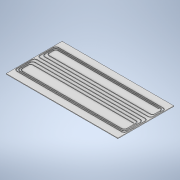
# Autodesk Inventor part: coil_layer
Saved by Autodesk Inventor 2021 (Build 250183000, 183)
## iProperties
Created: 2021-02-03
Part Number: coil_layer
Material: Generic
Document SubType Name: Modeling
Designer: User
Density: 1 g/cm^3
Appearance: Default
Author: User
Autodesk Inventor part; units mm, degrees
ref_plane "YZ Plane" through (0, 0, 0) normal (1, 0, 0) x (0, 1, 0)
ref_plane "XZ Plane" through (0, 0, 0) normal (0, 1, 0) x (-1, 0, 0)
ref_plane "XY Plane" through (0, 0, 0) normal (0, 0, 1) x (1, 0, 0)
sketch "Sketch1" plane through (0, 0, 0) normal (0, 1, 0) x (-1, 0, 0)
  line L0 (-17.9221, -19.934) -> (-497.9003, -19.934)
  line L1 (-517.9003, 3.6211) -> (-517.9003, 130.008)
  line L2 (-498.4559, 150) -> (251.5573, 150)
  line L3 (272.0997, 130.0022) -> (272.0997, 30.0874)
  line L4 (-18.4221, -15.434) -> (-497.9003, -15.434)
  line L5 (-513.4003, 3.3566) -> (-513.4003, 129.9936)
  line L6 (-498.4133, 145.5) -> (251.5937, 145.5)
  line L7 (267.5997, 130.0175) -> (267.5997, 30.093)
  line L8 (251.5818, 7.666) -> (-487.4606, 7.666)
  line L9 (-503.9003, 29.6772) -> (-503.9003, 120.4936)
  line L10 (251.5679, 3.166) -> (-477.2003, 3.166)
  line L11 (-508.4003, 30.3457) -> (-508.4003, 120.508)
  line L12 (-488.9133, 136) -> (242.0937, 136)
  line L13 (-488.9559, 140.5) -> (242.0573, 140.5)
  line L14 (258.0997, 120.5175) -> (258.0997, 56.5584)
  line L15 (242.2252, 30.766) -> (-474.4003, 30.766)
  line L16 (262.5997, 120.5022) -> (262.5997, 56.5974)
  line L17 (242.1573, 26.266) -> (-474.4003, 26.266)
  line L18 (-494.4003, 56.1758) -> (-494.4003, 110.9936)
  line L19 (-479.4133, 126.5) -> (232.5937, 126.5)
  line L20 (248.5997, 111.0175) -> (248.5997, 81.7203)
  line L21 (226.7413, 53.866) -> (-488.9221, 53.866)
  line L22 (-498.9003, 56.8436) -> (-498.9003, 111.008)
  line L23 (-479.4559, 131) -> (232.5573, 131)
  line L24 (253.0997, 111.0022) -> (253.0997, 83.0316)
  line L25 (226.7413, 49.366) -> (-488.9221, 49.366)
  line L26 (-122.9221, 150) -> (-122.9221, -150) construction
  line L27 (-18.9221, -15.434) -> (252.6121, -15.434)
  line L28 (271.0123, -33.8341) -> (271.0123, -129.4993)
  line L29 (251.5773, -149.4789) -> (-498.4319, -149.4789)
  line L30 (-518.377, -129.4966) -> (-518.377, -58.4688)
  line L31 (-18.9221, -19.934) -> (252.6121, -19.934)
  line L32 (266.5123, -33.8341) -> (266.5123, -129.4991)
  line L33 (251.5771, -144.9789) -> (-498.4273, -144.9789)
  line L34 (-498.449, -38.534) -> (242.0875, -38.534)
  line L35 (262.0712, -58.5177) -> (262.0712, -119.9846)
  line L36 (242.0769, -139.9789) -> (-488.9319, -139.9789)
  line L37 (-513.877, -129.4966) -> (-513.877, -58.4772)
  line L38 (-498.4397, -43.034) -> (242.0875, -43.034)
  line L39 (257.5712, -58.5177) -> (257.5712, -119.9846)
  line L40 (242.0769, -135.4789) -> (-488.9272, -135.4789)
  line L41 (-504.377, -119.9952) -> (-504.377, -84.5371)
  line L42 (-508.877, -119.9952) -> (-508.877, -84.9593)
  line L43 (-488.877, -61.634) -> (232.6078, -61.634)
  line L44 (252.6078, -84.9536) -> (252.6078, -110.5)
  line L45 (-488.877, -66.134) -> (232.6078, -66.134)
  line L46 (248.1078, -94.2732) -> (248.1078, -110.5)
  line L47 (232.5783, -125.9789) -> (-488.9221, -125.9789)
  line L48 (232.5775, -130.4789) -> (-488.9221, -130.4789)
  line L49 (-522.9003, 200.5211) -> (277.0997, 200.5211)
  arc A0 (251.5773, -149.4789) -> (271.0123, -129.4993) centre (251.2071, -129.6765) ccw
  arc A1 (251.5771, -144.9789) -> (266.5123, -129.4991) centre (251.2071, -129.6772) ccw
  arc A2 (242.0769, -135.4789) -> (257.5712, -119.9846) centre (242.0769, -119.9846) ccw
  arc A3 (242.0769, -139.9789) -> (262.0712, -119.9846) centre (242.0769, -119.9846) ccw
  arc A4 (232.5775, -130.4789) -> (252.6078, -110.5) centre (232.6051, -110.4763) ccw
  arc A5 (232.5783, -125.9789) -> (248.1078, -110.5) centre (232.6051, -110.4763) ccw
  line L50 (266.0656, -58.5177) -> (242.0875, -58.5177) construction
  line L51 (242.0875, -58.5177) -> (242.0875, -27) construction
  arc A6 (257.5712, -58.5177) -> (242.0875, -43.034) centre (242.0875, -58.5177) ccw
  arc A7 (262.0712, -58.5177) -> (242.0875, -38.534) centre (242.0875, -58.5177) ccw
  line L52 (252.6121, -3.7302) -> (252.6121, -33.8341) construction
  line L53 (252.6121, -33.8341) -> (272.6377, -33.8341) construction
  arc A8 (266.5123, -33.8341) -> (252.6121, -19.934) centre (252.6121, -33.8341) ccw
  arc A9 (271.0123, -33.8341) -> (252.6121, -15.434) centre (252.6121, -33.8341) ccw
  arc A10 (-518.377, -129.4966) -> (-498.4319, -149.4789) centre (-498.3932, -129.4952) ccw
  arc A11 (-513.877, -129.4966) -> (-498.4273, -144.9789) centre (-498.3932, -129.4952) ccw
  arc A12 (-508.877, -119.9952) -> (-488.9319, -139.9789) centre (-488.8932, -119.9952) ccw
  line L54 (-488.9221, -130.4789) -> (-488.9221, -125.9789)
  arc A13 (-504.377, -119.9952) -> (-488.9272, -135.4789) centre (-488.8932, -119.9952) ccw
  arc A14 (-498.4397, -43.034) -> (-513.877, -58.4772) centre (-498.3717, -58.5393) ccw
  arc A15 (-498.449, -38.534) -> (-518.377, -58.4688) centre (-498.3717, -58.5393) ccw
  line L55 (-488.9221, 49.366) -> (-488.9221, 53.866)
  arc A16 (-479.4133, 126.5) -> (-494.4003, 110.9936) centre (-479.0257, 111.1296) ccw
  arc A17 (-479.4559, 131) -> (-498.9003, 111.008) centre (-479.0257, 111.1296) ccw
  arc A18 (-488.9133, 136) -> (-503.9003, 120.4936) centre (-488.5257, 120.6296) ccw
  arc A19 (-488.9559, 140.5) -> (-508.4003, 120.508) centre (-488.5257, 120.6296) ccw
  arc A20 (-498.4133, 145.5) -> (-513.4003, 129.9936) centre (-498.0257, 130.1296) ccw
  arc A21 (-498.4559, 150) -> (-517.9003, 130.008) centre (-498.0257, 130.1296) ccw
  arc A22 (248.5997, 111.0175) -> (232.5937, 126.5) centre (232.9624, 110.8664) ccw
  arc A23 (253.0997, 111.0022) -> (232.5573, 131) centre (232.9624, 110.8664) ccw
  arc A24 (258.0997, 120.5175) -> (242.0937, 136) centre (242.4624, 120.3664) ccw
  arc A25 (262.5997, 120.5022) -> (242.0573, 140.5) centre (242.4624, 120.3664) ccw
  arc A26 (267.5997, 130.0175) -> (251.5937, 145.5) centre (251.9624, 129.8664) ccw
  arc A27 (272.0997, 130.0022) -> (251.5573, 150) centre (251.9624, 129.8664) ccw
  line L56 (-522.9003, -199.4789) -> (-522.9003, 200.5211)
  line L57 (267.5997, 30.093) -> (267.5997, 7.666) construction
  line L58 (267.5997, 7.666) -> (251.5818, 7.666) construction
  line L59 (242.1573, 26.266) -> (242.5997, 26.266) construction
  line L60 (262.5997, 26.266) -> (262.5997, 56.5974) construction
  line L61 (258.0997, 56.5584) -> (258.0997, 42.8204) construction
  line L62 (233.0997, 49.366) -> (253.0997, 49.366) construction
  line L63 (253.0997, 49.366) -> (253.0997, 83.0316) construction
  line L64 (248.5997, 81.7203) -> (248.5997, 53.866) construction
  line L65 (248.5997, 53.866) -> (232.2009, 53.866) construction
  line L66 (-494.4003, 56.1758) -> (-494.4003, 46.266) construction
  line L67 (-478.9003, 30.766) -> (-477.2003, 30.766) construction
  line L68 (-479.5767, 26.266) -> (-498.9003, 26.266) construction
  line L69 (-498.9003, 49.366) -> (-498.9003, 56.8436) construction
  line L70 (-487.4606, 7.666) -> (-503.9003, 7.666) construction
  line L71 (-503.9003, 29.6772) -> (-503.9003, 7.666) construction
  line L72 (-508.4003, 30.3457) -> (-508.4003, 23.166) construction
  line L73 (-508.4003, 3.166) -> (-489.0292, 3.166) construction
  line L74 (-498.4417, -15.434) -> (-513.4003, -15.434) construction
  line L75 (-517.9003, -19.934) -> (-498.4419, -19.934) construction
  line L76 (248.1078, -84.54) -> (248.1078, -66.134) construction
  line L77 (248.1078, -66.134) -> (232.6078, -66.134) construction
  line L78 (232.6078, -61.634) -> (252.6078, -61.634) construction
  line L79 (252.6078, -61.634) -> (252.6078, -84.9536) construction
  line L80 (-488.877, -61.634) -> (-508.877, -61.634) construction
  line L81 (-508.877, -61.634) -> (-508.877, -84.9593) construction
  line L82 (-488.877, -66.134) -> (-504.377, -66.134) construction
  line L83 (-504.377, -66.134) -> (-504.377, -84.5371) construction
  line L84 (-508.877, -61.634) -> (-508.877, -84.9593) construction
  line L85 (-498.9003, 26.266) -> (-488.9221, 26.266) construction
  line L86 (-478.9003, 26.266) -> (-478.9003, 46.266) construction
  line L87 (-478.9003, 46.266) -> (-498.9003, 46.266) construction
  line L88 (-494.4003, 50.766) -> (-494.4003, 46.266) construction
  line L89 (-474.4003, 30.766) -> (-474.4003, 26.266) construction
  arc A28 (-498.9003, 46.266) -> (-478.9003, 26.266) centre (-478.9003, 46.266) ccw
  arc A29 (-494.4003, 46.266) -> (-478.9003, 30.766) centre (-478.9003, 46.266) ccw
  line L90 (-498.9003, 56.8436) -> (-498.9003, 46.266)
  line L91 (-494.4003, 56.1758) -> (-494.4003, 46.266)
  line L92 (-478.9003, 30.766) -> (-474.4003, 30.766)
  line L93 (-478.9003, 26.266) -> (-474.4003, 26.266)
  line L94 (-488.4003, 3.166) -> (-488.4003, 23.166) construction
  line L95 (-488.4003, 23.166) -> (-508.4003, 23.166) construction
  arc A30 (-503.9003, 23.166) -> (-488.4003, 7.666) centre (-488.4003, 23.166) ccw
  line L96 (-488.4003, 7.666) -> (-487.4606, 7.666)
  line L97 (-477.2003, 9.3706) -> (-477.2003, 0.2696) construction
  arc A31 (-508.4003, 23.166) -> (-488.4003, 3.166) centre (-488.4003, 23.166) ccw
  line L98 (-508.4003, 30.3457) -> (-508.4003, 23.166)
  line L99 (-503.9003, 29.6772) -> (-503.9003, 23.166)
  line L100 (-488.4003, 3.166) -> (-477.2003, 3.166)
  line L101 (226.7413, 56.1758) -> (226.7413, 43.6622) construction
  arc A32 (233.0997, 53.866) -> (248.5997, 69.366) centre (233.0997, 69.366) ccw
  arc A33 (233.0997, 49.366) -> (253.0997, 69.366) centre (233.0997, 69.366) ccw
  line L102 (233.0997, 53.866) -> (226.7413, 53.866)
  line L103 (233.0997, 49.366) -> (226.7413, 49.366) construction
  line L104 (233.0997, 49.366) -> (226.7413, 49.366)
  line L105 (248.5997, 69.366) -> (248.5997, 81.7203)
  line L106 (253.0997, 83.0316) -> (253.0997, 69.366)
  line L107 (242.5997, 29.7117) -> (242.5997, 46.266) construction
  line L108 (242.5997, 46.266) -> (262.5997, 46.266) construction
  line L109 (242.1573, 26.266) -> (242.5997, 26.266) construction
  line L110 (242.1573, 26.266) -> (242.5997, 26.266)
  arc A34 (242.5997, 30.766) -> (258.0997, 46.266) centre (242.5997, 46.266) ccw
  arc A35 (242.5997, 26.266) -> (262.5997, 46.266) centre (242.5997, 46.266) ccw
  line L111 (258.0997, 46.266) -> (258.0997, 56.5584)
  line L112 (262.5997, 56.5974) -> (262.5997, 46.266)
  line L113 (242.2252, 30.766) -> (242.5997, 30.766)
  arc A36 (252.0997, 7.666) -> (267.5997, 23.166) centre (252.0997, 23.166) ccw
  line L114 (252.0997, 7.666) -> (251.5818, 7.666)
  line L115 (267.5997, 23.166) -> (267.5997, 30.093)
  arc A37 (252.0997, 3.166) -> (272.0997, 23.166) centre (252.0997, 23.166) ccw
  line L116 (251.5679, 3.166) -> (252.0997, 3.166)
  line L117 (272.0997, 23.166) -> (272.0997, 30.0874)
  arc A38 (-513.4003, 0.066) -> (-497.9003, -15.434) centre (-497.9003, 0.066) ccw
  arc A39 (-517.9003, 0.066) -> (-497.9003, -19.934) centre (-497.9003, 0.066) ccw
  line L118 (-517.9003, 0.066) -> (-517.9003, 3.6211)
  line L119 (-513.4003, 3.3566) -> (-513.4003, 0.066)
  line L120 (232.6078, -50.9214) -> (232.6078, -81.634) construction
  line L121 (232.6078, -81.634) -> (253.5598, -81.634) construction
  arc A40 (252.6078, -81.634) -> (232.6078, -61.634) centre (232.6078, -81.634) ccw
  arc A41 (248.1078, -81.634) -> (232.6078, -66.134) centre (232.6078, -81.634) ccw
  line L122 (252.6078, -81.634) -> (252.6078, -84.9536)
  line L123 (248.1078, -81.634) -> (248.1078, -94.2732)
  line L124 (-522.4266, -81.634) -> (-488.877, -81.634) construction
  line L125 (-488.877, -81.634) -> (-488.877, -54.4584) construction
  arc A42 (-488.877, -61.634) -> (-508.877, -81.634) centre (-488.877, -81.634) ccw
  arc A43 (-488.877, -66.134) -> (-504.377, -81.634) centre (-488.877, -81.634) ccw
  line L126 (-508.877, -81.634) -> (-508.877, -84.9593)
  line L127 (-504.377, -81.634) -> (-504.377, -84.5371)
  line L128 (-595.5051, -6.134) -> (317.0651, -6.134) construction
  line L129 (-522.9003, -199.4789) -> (277.0997, -199.4789) construction
  line L130 (277.0997, -199.4789) -> (277.0997, 200.5211) construction
  line L131 (-522.9003, -199.4789) -> (277.0997, -199.4789)
  line L132 (277.0997, 200.5211) -> (277.0997, -199.4789)
  point P0 (-228.9877, 0)
  point P1 (257.5779, -125.9789)
  point P2 (257.5712, -58.5177)
  dimension "d2" = 4.5
  dimension "d3" = 4.5
  dimension "d4" = 4.5
  dimension "d5" = 5
  dimension "d6" = 5
  dimension "d7" = 4.5
  dimension "d8" = 4.5
  dimension "d9" = 4.5
  dimension "d10" = 5
  dimension "d11" = 790
  dimension "d12" = 18.6
  dimension "d13" = 4.5
  dimension "d14" = 4.5
  dimension "d15" = 18.6
  dimension "d16" = 5
  dimension "d17" = 5
  dimension "d18" = 4.5
  dimension "d19" = 5
  dimension "d20" = 18.6
  dimension "d21" = 4.5
  dimension "d22" = 4.5
  dimension "d23" = 4.5
  dimension "d30" = 4.5
  dimension "d31" = 4.5
  dimension "d32" = 4.5
  dimension "d34" = 500
  dimension "d35" = 4.5
  dimension "d36" = 4.5
  dimension "d38" = 4.5
  dimension "d39" = 18.6
  dimension "d40" = 4.5
  dimension "d41" = 5
  dimension "d42" = 4.5
  dimension "d43" = 4.5
  dimension "d44" = 4.5
  dimension "d46" = 18.6
  dimension "d47" = 5
  dimension "d48" = 4.5
  dimension "d49" = 5
  dimension "d80" = 4.5
  dimension "d81" = 0
  dimension "d254" = 9.3
  dimension "d259" = 50
  dimension "d261" = 400
  constraints: 266 end point, 90 point on circle, 52 perpendicular, 44 centre point, 33 point on line, 28 coincident, 24 horizontal, 20 vertical, 16 collinear, 11 parallel, 1 tangent
  measures "d2" distance between parallel lines of L1 L5
  measures "d3" distance between parallel lines of L2 L6
  measures "d4" distance between parallel lines of L7 L3
  measures "d5" distance between parallel lines of L13 L6
  measures "d6" distance between parallel lines of L5 L11
  measures "d7" distance between parallel lines of L10 L8
  measures "d8" distance between parallel lines of L14 L16
  measures "d9" distance between parallel lines of L13 L12
  measures "d10" distance between parallel lines of L16 L7
  measures "d11" distance between parallel lines of L1 L3
  measures "d12" distance between parallel lines of L4 L10
  measures "d13" distance between parallel lines of L11 L9
  measures "d14" distance between parallel lines of L17 L15
  measures "d15" distance between parallel lines of L8 L17
  measures "d16" distance between parallel lines of L12 L23
  measures "d17" distance between parallel lines of L9 L22
  measures "d18" distance between parallel lines of L23 L19
  measures "d19" distance between parallel lines of L24 L14
  measures "d20" distance between parallel lines of L15 L25
  measures "d21" distance between parallel lines of L24 L20
  measures "d22" distance between parallel lines of L25 L21
  measures "d23" distance between parallel lines of L22 L18
  measures "d30" distance between parallel lines of L31 L27
  measures "d31" distance between parallel lines of L32 L28
  measures "d32" distance between parallel lines of L29 L33
  measures "d34" distance from line of point (-228.988, 0) L28
  measures "d35" distance between parallel lines of L30 L37
  measures "d36" distance between parallel lines of L39 L35
  measures "d38" distance between parallel lines of L34 L38
  measures "d39" distance between parallel lines of L34 L31
  measures "d40" distance between parallel lines of L36 L40
  measures "d41" distance between parallel lines of L33 L36
  measures "d42" distance between parallel lines of L42 L41
  measures "d43" distance between parallel lines of L43 L45
  measures "d44" distance between parallel lines of L46 L44
  measures "d46" distance between parallel lines of L43 L38
  measures "d47" distance between parallel lines of L37 L42
  measures "d48" distance between parallel lines of L48 L47
  measures "d49" distance between parallel lines of L40 L48
  measures "d80" distance between parallel lines of L4 L0
  measures "d81" distance between parallel lines of L0 L31
  measures "d254" distance between parallel lines of L10 L128
  measures "d259" distance between parallel lines of L129 L29
  measures "d261" distance of L49.end L129.end
extrude "Extrusion7" add sketch "Sketch1" along normal blind 4.5
equation "\"d6\" = d26"
equation "\"d10\" = d26"
equation "\"d16\" = d26"
equation "\"d19\" = d25"
equation "\"d34\" = 0.5 * d52"
equation "\"d41\" = d53"
equation "\"d47\" = d53"
equation "\"d49\" = d53"
equation "\"d25\" = 5"
equation "\"d26\" = 5"
equation "\"d28\" = -1.2 * d25 + 0.2 * d29"
equation "\"d51\" = 5"
equation "\"d53\" = 5"
equation "\"d54\" = -1.2 * d51 + 0.2 * d55"
equation "\"d29\" = 140"
equation "\"d55\" = 140"
equation "\"d52\" = 1000"
body "Solid5"
